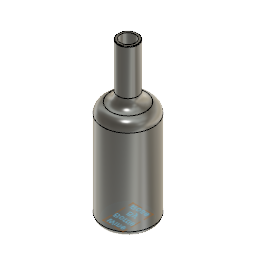
Wine Bottle v1 (Autodesk Fusion 360 design; units mm, degrees)
Autodesk Fusion 360 part; units mm, degrees
sketch "Sketch1" plane through (0, 0, 0) normal (0, 0, 1) x (1, 0, 0)
  circle A0 centre (0, 0) radius 50
  constraint coincident A0.centre origin
extrude "Extrude1" add sketch "Sketch1" along normal blind 200
sketch "Sketch2" plane through (0, 0, 200) normal (0, 0, 1) x (-1, 0, 0)
  circle A0 centre (0, 0) radius 50
  circle A1 centre (0, 0) radius 20
  constraint coincident A0.centre A1.centre
extrude "Extrude2" add sketch "Sketch2" along normal blind 110 contours A1
fillet "Fillet1" radius 20 1 faces at (39.7394, -3.4777, 200)
fillet "Fillet1" radius 10 1 edges at (-46.6164, -18.0808, 0)
sketch "Sketch3" plane through (0, 0, 310) normal (0, 0, 1) x (-1, 0, 0)
  circle A0 centre (0, 0) radius 20
  circle A1 centre (0, 0) radius 14.7761
  constraint coincident A0.centre A1.centre
extrude "Extrude3" add sketch "Sketch3" along normal blind 25 contours A1
fillet "Fillet2" radius 1 1 edges at (18.6465, 7.2323, 310)
torus "TorusPrimitive1" cut centre line diameter 80 section diameter 2 placed x (1, 0, 0) y (0, -1, 0) z (0, 0, -1) at (0, 0, 0)
extrude "Extrude4" cut 1 faces at (-0.6516, 3.6695, 335) along direction (0, 0, -1) blind 330
sketch "Sketch5" plane through (0, 0, 0) normal (1, 0, 0) x (0, 1, 0)
sketch "Sketch6" plane through (0, 0, 0) normal (0, 0, -1) x (1, 0, 0)
  circle A0 centre (0, 0) radius 39
  line L0 (-20, -30) -> (20, -30) construction
  line L1 (20, -30) -> (20, 30) construction
  line L2 (20, 30) -> (-20, 30) construction
  line L3 (-20, 30) -> (-20, -30) construction
  dimension "d17" = 10
